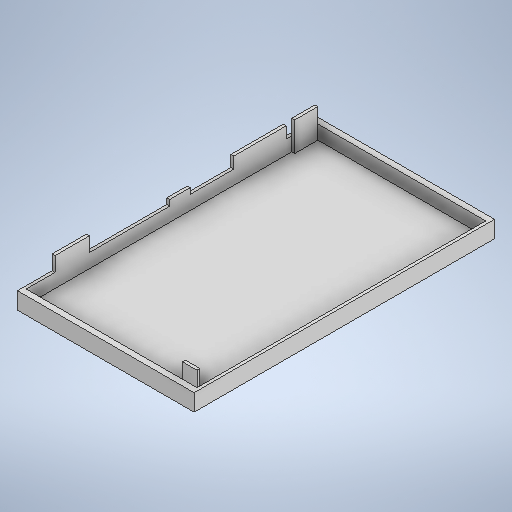
# Autodesk Inventor part: lid top
Saved by Autodesk Inventor 2025.2 (Build 292293000, 293)
## iProperties
Created: 2025-04-04
Part Number: lid top
Material: Generic
Document SubType Name: Modeling
Designer: joaki
Density: 1 g/cm^3
Appearance: Default
Author: joaki
Autodesk Inventor part; units mm, degrees
ref_plane "YZ Plane" through (0, 0, 0) normal (1, 0, 0) x (0, 1, 0)
ref_plane "XZ Plane" through (0, 0, 0) normal (0, 1, 0) x (-1, 0, 0)
ref_plane "XY Plane" through (0, 0, 0) normal (0, 0, 1) x (1, 0, 0)
sketch "Sketch1" plane through (0, 0, 0) normal (0, 1, 0) x (-1, 0, 0)
  line L0 (71.9808, 153.586) -> (11.2408, 153.586)
  line L1 (11.2408, 153.586) -> (11.2408, 50.288)
  line L2 (11.2408, 50.288) -> (71.9808, 50.288)
  line L3 (71.9808, 50.288) -> (71.9808, 153.586)
  point P0 (0, 0)
  dimension "d0" = 60.74
  dimension "d1" = 103.298
  constraints: 8 end point, 2 parallel, 1 horizontal, 1 perpendicular
  measures "d0" distance of L1.end L2.end
  measures "d1" distance of L0.end L1.end
extrude "Extrusion1" add sketch "Sketch1" along normal blind 1
sketch "Sketch2" plane through (0, 1, 0) normal (0, 1, 0) x (1, 0, 0)
  line L0 (-71.9808, -50.288) -> (-71.9808, -153.586) projected
  line L1 (-11.2408, -153.586) -> (-11.2408, -50.288) projected
  line L2 (-71.9808, -153.586) -> (-11.2408, -153.586)
  line L3 (-11.2408, -153.586) -> (-11.2408, -151.586)
  line L4 (-11.2408, -151.586) -> (-71.9808, -151.586)
  line L5 (-71.9808, -151.586) -> (-71.9808, -153.586)
  line L6 (-11.2408, -50.288) -> (-71.9808, -50.288) projected
  line L7 (-71.9808, -151.586) -> (-70.9808, -151.586)
  line L8 (-70.9808, -151.586) -> (-70.9808, -50.288)
  line L9 (-70.9808, -50.288) -> (-71.9808, -50.288)
  line L10 (-71.9808, -50.288) -> (-71.9808, -151.586)
  line L11 (-70.9808, -50.288) -> (-11.2408, -50.288)
  line L12 (-11.2408, -50.288) -> (-11.2408, -52.288)
  line L13 (-11.2408, -52.288) -> (-70.9808, -52.288)
  line L14 (-70.9808, -52.288) -> (-70.9808, -50.288)
  line L15 (-11.2408, -52.288) -> (-12.2408, -52.288)
  line L16 (-12.2408, -52.288) -> (-12.2408, -151.586)
  line L17 (-12.2408, -151.586) -> (-11.2408, -151.586)
  line L18 (-11.2408, -151.586) -> (-11.2408, -52.288)
  point P0 (0, 0)
  dimension "d4" = 2
  dimension "d5" = 1
  dimension "d6" = 2
  dimension "d7" = 1
  constraints: 32 end point, 8 parallel, 4 horizontal, 4 perpendicular, 4 point on line
  measures "d4" distance between parallel lines of L4 L2
  measures "d5" distance between parallel lines of L0 L8
  measures "d6" distance between parallel lines of L6 L13
  measures "d7" distance between parallel lines of L18 L16
extrude "Extrusion2" add sketch "Sketch2" along normal blind 4.8 contours L6 L8 L4 L0 | L4 L1 L2 L0 | L6 L1 L13 L8 | L16 L13 L1 L4
sketch "Sketch3" plane through (0, 5.8, 0) normal (0, 1, 0) x (1, 0, 0)
  line L0 (-71.9808, -50.288) -> (-71.9808, -153.586) projected
  line L1 (-71.9808, -153.586) -> (-71.9808, -141.686)
  line L2 (-70.9808, -52.288) -> (-70.9808, -151.586) projected
  line L3 (-71.9808, -141.686) -> (-70.9808, -141.686)
  line L4 (-70.9808, -141.686) -> (-70.9808, -129.786)
  line L5 (-70.9808, -129.786) -> (-71.9808, -129.786)
  line L6 (-71.9808, -129.786) -> (-71.9808, -141.686)
  point P0 (0, 0)
  point P1 (-71.4808, -129.786)
  point P2 (-71.4808, -141.686)
  dimension "d18" = 11.9
  dimension "d19" = 11.9
  constraints: 10 end point, 2 midpoint, 2 parallel, 2 point on line, 1 horizontal, 1 perpendicular
  measures "d18" distance of L0.end L1.end
  measures "d19" distance of point (-71.481, -129.786) point (-71.481, -141.686)
extrude "Extrusion3" add sketch "Sketch3" along normal blind 5
sketch "Sketch4" plane through (0, 5.8, 0) normal (0, 1, 0) x (1, 0, 0)
  line L0 (-71.9808, -129.786) -> (-71.9808, -116.586)
  line L1 (-71.9808, -50.288) -> (-71.9808, -129.786) projected
  line L2 (-70.9808, -129.786) -> (-70.9808, -52.288) projected
  line L3 (-71.9808, -116.586) -> (-70.9808, -116.586)
  line L4 (-70.9808, -116.586) -> (-70.9808, -110.586)
  line L5 (-70.9808, -110.586) -> (-71.9808, -110.586)
  line L6 (-71.9808, -110.586) -> (-71.9808, -116.586)
  line L7 (-71.9808, -110.586) -> (-71.9808, -102.186)
  line L8 (-71.9808, -102.186) -> (-70.9808, -102.186)
  line L9 (-70.9808, -102.186) -> (-70.9808, -95.186)
  line L10 (-70.9808, -95.186) -> (-71.9808, -95.186)
  line L11 (-71.9808, -95.186) -> (-71.9808, -102.186)
  point P0 (0, 0)
  point P1 (-71.4808, -110.586)
  point P2 (-71.4808, -116.586)
  point P3 (-71.4808, -95.186)
  point P4 (-71.4808, -102.186)
  dimension "d22" = 13.2
  dimension "d23" = 6
  dimension "d24" = 8.4
  dimension "d25" = 7
  constraints: 20 end point, 4 midpoint, 4 parallel, 4 point on line, 2 horizontal, 2 perpendicular
  measures "d22" distance of L0.start L0.end
  measures "d23" distance of point (-71.481, -110.586) point (-71.481, -116.586)
  measures "d24" distance of L5.end L7.end
  measures "d25" distance of point (-71.481, -95.186) point (-71.481, -102.186)
extrude "Extrusion4" add sketch "Sketch4" along normal blind 2 contours L10 L2 L8 L1
sketch "Sketch5" plane through (0, 5.8, 0) normal (0, 1, 0) x (1, 0, 0)
  line L0 (-71.9808, -95.186) -> (-71.9808, -102.186) projected
  line L1 (-71.9808, -95.186) -> (-71.9808, -80.186)
  line L2 (-71.9808, -50.288) -> (-71.9808, -95.186) projected
  line L3 (-70.9808, -95.186) -> (-70.9808, -52.288) projected
  line L4 (-71.9808, -80.186) -> (-70.9808, -80.186)
  line L5 (-70.9808, -80.186) -> (-70.9808, -62.186)
  line L6 (-70.9808, -62.186) -> (-71.9808, -62.186)
  line L7 (-71.9808, -62.186) -> (-71.9808, -80.186)
  point P0 (0, 0)
  point P1 (-71.4808, -62.186)
  point P2 (-71.4808, -80.186)
  dimension "d28" = 15
  dimension "d29" = 18
  constraints: 10 end point, 2 midpoint, 2 parallel, 2 point on line, 1 horizontal, 1 perpendicular
  measures "d28" distance of L0.start L1.end
  measures "d29" distance of point (-71.481, -62.186) point (-71.481, -80.186)
extrude "Extrusion5" add sketch "Sketch5" along normal blind 3.9
sketch "Sketch6" plane through (0, 1, 0) normal (0, 1, 0) x (1, 0, 0)
  line L0 (-70.9808, -62.186) -> (-70.9808, -52.288) projected
  line L1 (-70.9808, -52.288) -> (-69.9808, -52.288)
  line L2 (-69.9808, -52.288) -> (-69.9808, -60.288)
  line L3 (-69.9808, -60.288) -> (-70.9808, -60.288)
  line L4 (-70.9808, -60.288) -> (-70.9808, -52.288)
  line L5 (-12.2408, -151.586) -> (-17.2408, -151.586)
  line L6 (-17.2408, -151.586) -> (-17.2408, -150.586)
  line L7 (-17.2408, -150.586) -> (-12.2408, -150.586)
  line L8 (-12.2408, -150.586) -> (-12.2408, -151.586)
  point P0 (0, 0)
  point P1 (-70.4808, -52.288)
  point P2 (-70.4808, -60.288)
  point P3 (-17.2408, -151.086)
  point P4 (-12.2408, -151.086)
  dimension "d32" = 1
  dimension "d33" = 8
  dimension "d34" = 1
  dimension "d35" = 5
  constraints: 16 end point, 4 midpoint, 4 parallel, 2 horizontal, 2 perpendicular
  measures "d32" distance between parallel lines of L0 L2
  measures "d33" distance of point (-70.481, -52.288) point (-70.481, -60.288)
  measures "d34" distance between parallel lines of L7 L5
  measures "d35" distance of point (-17.241, -151.086) point (-12.241, -151.086)
extrude "Extrusion6" add sketch "Sketch6" along normal blind 10
body "Solid1"
